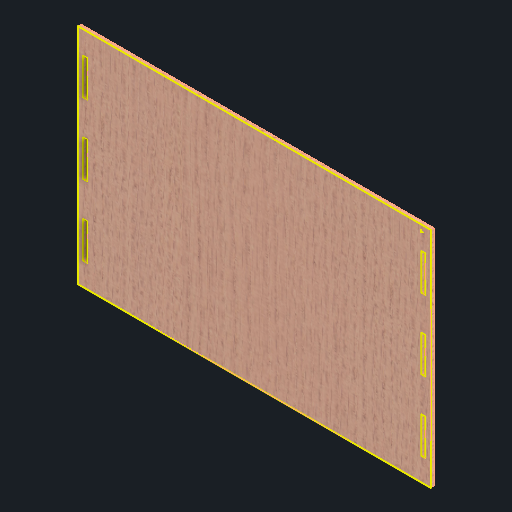
# Autodesk Inventor part: Stand Base
Saved by Autodesk Inventor 2025.2 (Build 292293000, 293)
## iProperties
Created: 2024-11-19
Part Number: Stand Base
Material: Wood (Oak)
Document SubType Name: Modeling
Designer: JL
Density: 0.76 g/cm^3
Appearance: White Oak - Natural Medium Gloss
Author: JL
Autodesk Inventor part; units mm, degrees
ref_plane "YZ Plane" through (0, 0, 0) normal (1, 0, 0) x (0, 1, 0)
ref_plane "XZ Plane" through (0, 0, 0) normal (0, 1, 0) x (-1, 0, 0)
ref_plane "XY Plane" through (0, 0, 0) normal (0, 0, 1) x (1, 0, 0)
ref_plane "Work Plane1" through (0, -46.6, 0) normal (0, 0, 1) x (1, 0, 0)
sketch "Sketch1" plane through (0, -46.6, 0) normal (0, 0, 1) x (1, 0, 0)
  line L0 (0, 31.0667) -> (0, 0) projected
  line L1 (0, 0) -> (3, 0) projected
  line L2 (3, 31.0667) -> (3, 0) projected
  line L3 (0, 31.0667) -> (3, 31.0667) projected
  line L4 (0, -31.0667) -> (0, -62.1333) projected
  line L5 (0, -62.1333) -> (3, -62.1333) projected
  line L6 (3, -31.0667) -> (3, -62.1333) projected
  line L7 (0, -31.0667) -> (3, -31.0667) projected
  line L8 (0, -93.2) -> (0, -124.2667) projected
  line L9 (0, -124.2667) -> (3, -124.2667) projected
  line L10 (3, -93.2) -> (3, -124.2667) projected
  line L11 (0, -93.2) -> (3, -93.2) projected
  line L12 (-297.2462, 31.0667) -> (-297.2462, 0) projected
  line L13 (-297.2462, 0) -> (-294.2462, 0) projected
  line L14 (-294.2462, 31.0667) -> (-294.2462, 0) projected
  line L15 (-297.2462, 31.0667) -> (-294.2462, 31.0667) projected
  line L16 (-297.2462, -31.0667) -> (-297.2462, -62.1333) projected
  line L17 (-297.2462, -62.1333) -> (-294.2462, -62.1333) projected
  line L18 (-294.2462, -31.0667) -> (-294.2462, -62.1333) projected
  line L19 (-297.2462, -31.0667) -> (-294.2462, -31.0667) projected
  line L20 (-297.2462, -93.2) -> (-297.2462, -124.2667) projected
  line L21 (-297.2462, -124.2667) -> (-294.2462, -124.2667) projected
  line L22 (-294.2462, -93.2) -> (-294.2462, -124.2667) projected
  line L23 (-297.2462, -93.2) -> (-294.2462, -93.2) projected
  line L24 (3, 46.6) -> (3, 31.0667) projected
  line L25 (-297.2462, -124.2667) -> (-297.2462, -139.8) projected
  line L26 (8, 51.6) -> (-302.2462, 51.6)
  line L27 (-302.2462, 51.6) -> (-302.2462, -144.8)
  line L28 (-302.2462, -144.8) -> (8, -144.8)
  line L29 (8, -144.8) -> (8, 51.6)
  line L30 (-293.9962, 31.3167) -> (-293.9962, -0.25)
  line L31 (-293.9962, -0.25) -> (-297.4962, -0.25)
  line L32 (-297.4962, -0.25) -> (-297.4962, 31.3167)
  line L33 (-297.4962, 31.3167) -> (-293.9962, 31.3167)
  line L34 (-293.9962, -30.8167) -> (-293.9962, -62.3833)
  line L35 (-293.9962, -62.3833) -> (-297.4962, -62.3833)
  line L36 (-297.4962, -62.3833) -> (-297.4962, -30.8167)
  line L37 (-297.4962, -30.8167) -> (-293.9962, -30.8167)
  line L38 (-293.9962, -124.5167) -> (-297.4962, -124.5167)
  line L39 (-297.4962, -124.5167) -> (-297.4962, -92.95)
  line L40 (-297.4962, -92.95) -> (-293.9962, -92.95)
  line L41 (-293.9962, -92.95) -> (-293.9962, -124.5167)
  line L42 (3.25, 31.3167) -> (3.25, -0.25)
  line L43 (3.25, -0.25) -> (-0.25, -0.25)
  line L44 (-0.25, -0.25) -> (-0.25, 31.3167)
  line L45 (-0.25, 31.3167) -> (3.25, 31.3167)
  line L46 (3.25, -30.8167) -> (3.25, -62.3833)
  line L47 (3.25, -62.3833) -> (-0.25, -62.3833)
  line L48 (-0.25, -62.3833) -> (-0.25, -30.8167)
  line L49 (-0.25, -30.8167) -> (3.25, -30.8167)
  line L50 (3.25, -92.95) -> (3.25, -124.5167)
  line L51 (3.25, -124.5167) -> (-0.25, -124.5167)
  line L52 (-0.25, -124.5167) -> (-0.25, -92.95)
  line L53 (-0.25, -92.95) -> (3.25, -92.95)
  point P0 (0, 46.6)
  dimension "d0" = 5
  dimension "d1" = 5
  dimension "d2" = 5
  dimension "d3" = 5
  dimension "d6" = 0.25
  dimension "d7" = 0.25
  dimension "d8" = 0.25
  dimension "d9" = 0.25
  dimension "d10" = 0.25
  dimension "d11" = 0.25
  constraints: 56 end point, 2 parallel, 1 horizontal, 1 perpendicular, 18 other
  measures "d0" distance between parallel lines of L29 L24
  measures "d1" distance from line of L26 L24.start
  measures "d2" distance between parallel lines of L27 L25
  measures "d3" distance from line of L28 L25.end
  measures "d6" distance between parallel lines of L15 L33
  measures "d7" distance between parallel lines of L19 L37
  measures "d8" distance between parallel lines of L21 L38
  measures "d9" distance between parallel lines of L3 L45
  measures "d10" distance between parallel lines of L7 L49
  measures "d11" distance between parallel lines of L11 L53
extrude "Extrusion1" add sketch "Sketch1" along normal blind 3 contours L29 L28 L27 L26
sketch "Sketch2" plane through (0, -46.6, 3) normal (0, 0, 1) x (1, 0, 0)
  line L0 (-302.2462, 51.6) -> (-302.2462, -144.8) projected
  line L1 (-302.2462, -144.8) -> (8, -144.8) projected
  line L2 (8, -144.8) -> (8, 51.6) projected
  line L3 (8, 51.6) -> (-302.2462, 51.6) projected
  line L4 (3.25, -92.95) -> (3.25, -124.5167) projected
  line L5 (3.25, -124.5167) -> (-0.25, -124.5167) projected
  line L6 (-0.25, -124.5167) -> (-0.25, -92.95) projected
  line L7 (-0.25, -92.95) -> (3.25, -92.95) projected
  line L8 (3.25, -30.8167) -> (3.25, -62.3833) projected
  line L9 (3.25, -62.3833) -> (-0.25, -62.3833) projected
  line L10 (-0.25, -62.3833) -> (-0.25, -30.8167) projected
  line L11 (-0.25, -30.8167) -> (3.25, -30.8167) projected
  line L12 (-293.9962, -30.8167) -> (-293.9962, -62.3833) projected
  line L13 (-293.9962, -62.3833) -> (-297.4962, -62.3833) projected
  line L14 (-297.4962, -62.3833) -> (-297.4962, -30.8167) projected
  line L15 (-297.4962, -30.8167) -> (-293.9962, -30.8167) projected
  line L16 (-293.9962, 31.3167) -> (-293.9962, -0.25) projected
  line L17 (-293.9962, -0.25) -> (-297.4962, -0.25) projected
  line L18 (-297.4962, -0.25) -> (-297.4962, 31.3167) projected
  line L19 (-297.4962, 31.3167) -> (-293.9962, 31.3167) projected
  line L20 (-0.25, -0.25) -> (-0.25, 31.3167) projected
  line L21 (-0.25, 31.3167) -> (3.25, 31.3167) projected
  line L22 (3.25, 31.3167) -> (3.25, -0.25) projected
  line L23 (3.25, -0.25) -> (-0.25, -0.25) projected
  line L24 (-293.9962, -92.95) -> (-293.9962, -124.5167) projected
  line L25 (-293.9962, -124.5167) -> (-297.4962, -124.5167) projected
  line L26 (-297.4962, -124.5167) -> (-297.4962, -92.95) projected
  line L27 (-297.4962, -92.95) -> (-293.9962, -92.95) projected
  point P0 (0, 46.6)
equation "\"d7\" = d6"
equation "\"d8\" = d6"
equation "\"d9\" = d6"
equation "\"d10\" = d6"
equation "\"d11\" = d6"
body "Solid1"
